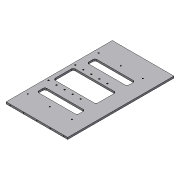
# Autodesk Inventor part: TL20240701-10110CV-001
Saved by Autodesk Inventor 2022.5 (Build 265521000, 521)
## iProperties
Category: DRIVE UNIT ASSY
Company: 현대 트랜시스(대유)
Created: 2023-04-10
Part Number: TL20240701-10110CV-001
Checked By: 김형민
Engr Approved By: 김시현
User Status: 1 x18
Material: SS400
Description: 0
Document SubType Name: Modeling
Mfg Approved By: 호상태
Designer: 박성규
Stock Number: 001
Density: 7.85 g/cm^3
Appearance: Painting-RAL7035
Mass: 36342.3 g
Surface Area: 8278.95 cm^2
Volume: 4629.59 cm^3
Project: SW PJT
DETAIL: Coveryor Assembly
M/C TITLE: CJ 제일제당 협동로봇 포장시스탬 PILOT 장비
PARTS NAME: Bracket
SPECIFICATION: TA20221101-CV200000-015
DocNumber: 221118_Standard_v1
Folder: .\
VDS_Category: 엔지니어링
PLATE_L: 794.000 mm
Detail Description: Processed products
Title: BASE
Subject: SW차종 시트조립라인
Author: 박성규
Revision Number: B
Autodesk Inventor part; units mm, degrees
ref_plane "YZ Plane" through (0, 0, 0) normal (1, 0, 0) x (0, 1, 0)
ref_plane "XZ Plane" through (0, 0, 0) normal (0, 1, 0) x (-1, 0, 0)
ref_plane "XY Plane" through (0, 0, 0) normal (0, 0, 1) x (1, 0, 0)
sketch "스케치9" plane through (0, 0, 0) normal (0, 0, 1) x (1, 0, 0)
  line L0 (-230, 7) -> (230, 7)
  line L1 (230, 7) -> (230, -7)
  line L2 (230, -7) -> (-230, -7)
  line L3 (-230, -7) -> (-230, 7)
  line L4 (-230, 7) -> (230, -7) construction
  line L5 (230, 7) -> (-230, -7) construction
  point P0 (0, 0)
  dimension "d40" = 460
  dimension "d41" = 14
  constraints: 12 end point, 2 midpoint, 2 parallel, 1 horizontal, 1 perpendicular
  measures "d40" distance of L0.start L0.end
  measures "d41" distance of L0.end L1.end
extrude "돌출4" add sketch "스케치9" along normal mid plane 794
sketch "스케치15" plane through (-230, 7, 397) normal (0, 1, 0) x (1, 0, 0)
  line L0 (0, 794) -> (0, 0) construction
  line L1 (30, 322) -> (350, 322)
  line L2 (350, 322) -> (350, 472)
  line L3 (350, 472) -> (30, 472)
  line L4 (30, 472) -> (30, 322)
  line L5 (30, 322) -> (350, 472) construction
  line L6 (350, 322) -> (30, 472) construction
  line L7 (50, 240) -> (350, 240)
  line L8 (350, 240) -> (350, 180)
  line L9 (350, 180) -> (50, 180)
  line L10 (50, 180) -> (50, 240)
  line L11 (50, 554) -> (350, 554)
  line L12 (350, 554) -> (350, 614)
  line L13 (350, 614) -> (50, 614)
  line L14 (50, 614) -> (50, 554)
  line L15 (460, 0) -> (0, 0) projected
  line L16 (0, 397) -> (460, 397) construction
  line L17 (460, 794) -> (460, 0) projected
  point P0 (230, 397)
  point P1 (190, 397)
  point P2 (190, 397)
  dimension "d120" = 50
  dimension "d122" = 180
  dimension "d123" = 60
  dimension "d129" = 320
  dimension "d130" = 30
  dimension "d131" = 150
  dimension "d136" = 300
  constraints: 30 end point, 6 parallel, 5 midpoint, 3 horizontal, 3 perpendicular, 2 point on line, 1 collinear, 1 horizontal alignment, 1 other
  measures "d120" distance between parallel lines of L10 L0
  measures "d122" distance between parallel lines of L9 L15
  measures "d123" distance between parallel lines of L7 L9
  measures "d129" distance of L1.start L1.end
  measures "d130" distance between parallel lines of L0 L4
  measures "d131" distance between parallel lines of L3 L1
  measures "d136" distance of L8.end L9.end
extrude "돌출6" cut sketch "스케치15" against normal through all
sketch "스케치12" plane through (-230, 7, 397) normal (0, 1, 0) x (1, 0, 0)
  line L0 (360, 662) -> (30, 662)
  line L1 (30, 662) -> (30, 132)
  line L2 (30, 132) -> (360, 132)
  line L3 (360, 132) -> (360, 662)
  line L4 (360, 662) -> (30, 132) construction
  line L5 (30, 662) -> (360, 132) construction
  line L6 (460, 0) -> (0, 0) projected
  line L7 (0, 794) -> (460, 794) projected
  line L8 (0, 794) -> (0, 0) projected
  point P0 (230, 397)
  point P1 (195, 397)
  point P2 (195, 397)
  point P3 (195, 397)
  point P4 (195, 132)
  point P5 (195, 662)
  dimension "d66" = 330
  dimension "d133" = 132
  dimension "d134" = 132
  dimension "d135" = 30
  constraints: 12 end point, 6 midpoint, 4 coincident, 2 parallel, 1 horizontal, 1 horizontal alignment, 1 perpendicular
  measures "d66" distance of L1.end L2.end
  measures "d133" distance between parallel lines of L6 L2
  measures "d134" distance between parallel lines of L0 L7
  measures "d135" distance between parallel lines of L1 L8
hole "구멍4" at (-200, 7, 265) at (-35, 7, 265) at (130, 7, 265) at (130, 7, -265) at (-35, 7, -265) at (-200, 7, -265) direction (0, -1, 0) diameter 8.376 end through all thread size "M10x1.5" class "6H" standard "ISO Metric profile"
sketch "스케치13" plane through (0, 0, 397) normal (0, 0, 1) x (1, 0, 0)
  line L0 (-230, -7) -> (230, -7) construction
  line L1 (-230, 7) -> (-230, -7) construction
  point P0 (0, 0)
  point P1 (-200, 0)
  point P2 (-100, 0)
  point P3 (0, 0)
  point P4 (100, 0)
  point P5 (200, 0)
  dimension "d76" = 30
  dimension "d77" = 7
  dimension "d78" = 100
  dimension "d79" = 100
  dimension "d80" = 100
  dimension "d81" = 100
  constraints: 4 horizontal alignment
  measures "d76" distance from line of L1 point (-200, 0)
  measures "d77" distance from line of L0 point (-200, 0)
  measures "d78" distance of point (-100, 0) point (-200, 0)
  measures "d79" distance of point (0, 0) point (-100, 0)
  measures "d80" distance of point (100, 0) point (0, 0)
  measures "d81" distance of point (100, 0) point (200, 0)
hole "구멍5" at (-200, 0, 397) at (-100, 0, 397) at (0, 0, 397) at (100, 0, 397) at (200, 0, 397) direction (0, 0, -1) diameter 6.647 depth 22.2 tip angle 118 thread size "M8x1.25" class "6H" standard "ISO Metric profile"
sketch "스케치14" plane through (0, 0, -397) normal (0, 0, -1) x (-1, 0, 0)
  circle A0 centre (-200, 0) radius 3.3235 construction
  circle A1 centre (-100, 0) radius 3.3235 construction
  circle A2 centre (0, 0) radius 3.3235 construction
  circle A3 centre (100, 0) radius 3.3235 construction
  circle A4 centre (200, 0) radius 3.3235 construction
  point P0 (0, 0)
  constraints: 5 coincident
hole "구멍6" at (200, 0, -397) at (100, 0, -397) at (0, 0, -397) at (-100, 0, -397) at (-200, 0, -397) direction (0, 0, 1) diameter 6.647 depth 22.2 tip angle 118 thread size "M8x1.25" class "6H" standard "ISO Metric profile"
sketch "스케치16" plane through (-230, 7, 397) normal (0, 1, 0) x (1, 0, 0)
  line L0 (0, 794) -> (0, 0) construction
  point P0 (230, 397)
  point P1 (20, 297)
  point P2 (140, 297)
  point P3 (200, 297)
  point P4 (200, 497)
  point P5 (140, 497)
  point P6 (20, 497)
  point P7 (0, 397)
  point P8 (80, 497)
  point P9 (80, 297)
  point P10 (260, 297)
  point P11 (260, 497)
  dimension "d137" = 20
  dimension "d138" = 200
  dimension "d139" = 100
  dimension "d140" = 60
  dimension "d141" = 60
  dimension "d142" = 60
  dimension "d143" = 60
  constraints: 8 horizontal alignment, 5 vertical alignment, 1 midpoint
  measures "d137" distance from line of point (20, 497) L0
  measures "d138" distance of point (20, 497) point (20, 297)
  measures "d139" vertical distance of point (20, 497) point (0, 397)
  measures "d140" distance of point (80, 497) point (20, 497)
  measures "d141" distance of point (140, 497) point (80, 497)
  measures "d142" distance of point (140, 497) point (200, 497)
  measures "d143" distance of point (260, 497) point (200, 497)
hole "구멍7" at (-210, 7, 100) at (-90, 7, 100) at (-30, 7, 100) at (-30, 7, -100) at (-90, 7, -100) at (-210, 7, -100) at (-150, 7, -100) at (-150, 7, 100) at (30, 7, 100) at (30, 7, -100) direction (0, -1, 0) diameter 10.106 end through all thread size "M12x1.75" class "6H" standard "ISO Metric profile"
fillet "Fillet3" radius 15 12 edges at (-180, 0, 157) (-180, 0, 217) (120, 0, 217) (120, 0, 157) (120, 0, 75) (-200, 0, 75) (-200, 0, -75) (120, 0, -75) (120, 0, -157) (120, 0, -217) (-180, 0, -157) (-180, 0, -217)
equation "\"d79\" = d78"
equation "\"d80\" = d79"
equation "\"d81\" = d80"
